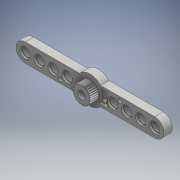
# Autodesk Inventor part: led-prop
Saved by Autodesk Inventor 2016 (Build 200138000, 138)
## iProperties
Created: 2016-11-01
Part Number: led-prop
Material: Generic
Document SubType Name: Modeling
Designer: Matt Ruffner
Density: 1 g/cm^3
Appearance: Default
Author: Matt Ruffner
Autodesk Inventor part; units mm, degrees
ref_plane "YZ Plane" through (0, 0, 0) normal (1, 0, 0) x (0, 1, 0)
ref_plane "XZ Plane" through (0, 0, 0) normal (0, 1, 0) x (-1, 0, 0)
ref_plane "XY Plane" through (0, 0, 0) normal (0, 0, 1) x (1, 0, 0)
sketch "Sketch1" plane through (0, 0, 0) normal (0, 1, 0) x (-1, 0, 0)
  circle A0 centre (24.5, 0) radius 5.05
  circle A1 centre (39.5, 0) radius 5.05
  circle A2 centre (54.5, 0) radius 5.05
  circle A3 centre (69.5, 0) radius 5.05
  circle A4 centre (-69.5, 0) radius 5.05
  circle A5 centre (-54.5, 0) radius 5.05
  circle A6 centre (-39.5, 0) radius 5.05
  circle A7 centre (-24.5, 0) radius 5.05
  line L0 (69.5, -10) -> (11.1803, -10)
  line L1 (69.5, 10) -> (11.1803, 10)
  arc A8 (69.5, -10) -> (69.5, 10) centre (69.5, 0) ccw
  line L2 (-69.5, -10) -> (-11.1803, -10)
  arc A9 (-69.5, 10) -> (-69.5, -10) centre (-69.5, 0) ccw
  line L3 (-69.5, 10) -> (-11.1803, 10)
  arc A10 (11.1803, 10) -> (-11.1803, 10) centre (0, 0) ccw
  arc A11 (-11.1803, -10) -> (11.1803, -10) centre (0, 0) ccw
  dimension "d1" = 10.1
  dimension "d2" = 10.1
  dimension "d3" = 10.1
  dimension "d4" = 10.1
  dimension "d5" = 24.5
  dimension "d6" = 15
  dimension "d7" = 15
  dimension "d8" = 15
  dimension "d11" = 360
  dimension "d16" = 360
  constraints: 12 centre point, 8 end point, 8 point on circle, 2 coincident, 2 horizontal, 34 other
  measures "d1" diameter of A0
  measures "d2" diameter of A1
  measures "d3" diameter of A2
  measures "d4" diameter of A3
  measures "d5" distance of A0.centre point (0, 0)
  measures "d6" distance of A1.centre A0.centre
  measures "d7" distance of A2.centre A1.centre
  measures "d8" distance of A3.centre A2.centre
extrude "Extrusion1" add sketch "Sketch1" along normal blind 9
sketch "Sketch2" plane through (0, 0, 0) normal (0, -1, 0) x (1, 0, 0)
  circle A0 centre (-69.5, 0) radius 5.05 projected
  circle A1 centre (-54.5, 0) radius 5.05 projected
  circle A2 centre (-39.5, 0) radius 5.05 projected
  circle A3 centre (-24.5, 0) radius 5.05 projected
  circle A4 centre (24.5, 0) radius 5.05 projected
  circle A5 centre (39.5, 0) radius 5.05 projected
  circle A6 centre (54.5, 0) radius 5.05 projected
  circle A7 centre (69.5, 0) radius 5.05 projected
  circle A8 centre (-69.5, 0) radius 5.6
  circle A9 centre (-54.5, 0) radius 5.6
  circle A10 centre (-39.5, 0) radius 5.6
  circle A11 centre (-24.5, 0) radius 5.6
  circle A12 centre (24.5, 0) radius 5.6
  circle A13 centre (39.5, 0) radius 5.6
  circle A14 centre (54.5, 0) radius 5.6
  circle A15 centre (69.5, 0) radius 5.6
  point P0 (0, 0)
  dimension "d20" = 11.2
  dimension "d21" = 11.2
  dimension "d22" = 11.2
  dimension "d23" = 11.2
  dimension "d24" = 11.2
  dimension "d25" = 11.2
  dimension "d26" = 11.2
  dimension "d27" = 11.2
  constraints: 8 centre point, 8 coincident
  measures "d20" diameter of A8
  measures "d21" diameter of A9
  measures "d22" diameter of A10
  measures "d23" diameter of A11
  measures "d24" diameter of A12
  measures "d25" diameter of A13
  measures "d26" diameter of A14
  measures "d27" diameter of A15
extrude "Extrusion2" cut sketch "Sketch2" against normal blind 2
sketch "Sketch4" plane through (0, 0, 0) normal (0, -1, 0) x (1, 0, 0)
  circle A0 centre (0, 0) radius 4.1
  circle A1 centre (0, 0) radius 9.75
  line L0 (0.0369, 9.7499) -> (-0.7015, 8.471)
  line L1 (0.0369, 9.7499) -> (1.3056, 9.7499) construction
  line L2 (0.0369, 9.7499) -> (0.7792, 8.4642)
  line L3 (0.0369, 9.7499) -> (1.4839, 9.7499) construction
  line L4 (-1.8659, 9.5698) -> (-2.3406, 8.1714)
  line L5 (-1.8659, 9.5698) -> (-0.887, 8.4536)
  line L6 (-3.697, 9.0219) -> (-3.8898, 7.5577)
  line L7 (-3.697, 9.0219) -> (-2.5192, 8.1181)
  line L8 (-5.3861, 8.1273) -> (-5.2895, 6.6537)
  line L9 (-5.3861, 8.1273) -> (-4.0546, 7.4706)
  line L10 (-6.8681, 6.9203) -> (-6.4859, 5.4939)
  line L11 (-6.8681, 6.9203) -> (-5.4341, 6.5361)
  line L12 (-8.0863, 5.4475) -> (-7.4331, 4.123)
  line L13 (-8.0863, 5.4475) -> (-6.6048, 5.3504)
  line L14 (-8.9936, 3.7652) -> (-8.0946, 2.5936)
  line L15 (-8.9936, 3.7652) -> (-7.5217, 3.959)
  line L16 (-9.5554, 1.9383) -> (-8.4451, 0.9646)
  line L17 (-9.5554, 1.9383) -> (-8.1496, 2.4155)
  line L18 (-9.7499, 0.0369) -> (-8.471, -0.7015)
  line L19 (-9.7499, 0.0369) -> (-8.4642, 0.7792)
  line L20 (-9.5698, -1.8659) -> (-8.1714, -2.3406)
  line L21 (-9.5698, -1.8659) -> (-8.4536, -0.887)
  line L22 (-9.0219, -3.697) -> (-7.5577, -3.8898)
  line L23 (-9.0219, -3.697) -> (-8.1181, -2.5192)
  line L24 (-8.1273, -5.3861) -> (-6.6537, -5.2895)
  line L25 (-8.1273, -5.3861) -> (-7.4706, -4.0546)
  line L26 (-6.9203, -6.8681) -> (-5.4939, -6.4859)
  line L27 (-6.9203, -6.8681) -> (-6.5361, -5.4341)
  line L28 (-5.4475, -8.0863) -> (-4.123, -7.4331)
  line L29 (-5.4475, -8.0863) -> (-5.3504, -6.6048)
  line L30 (-3.7652, -8.9936) -> (-2.5936, -8.0946)
  line L31 (-3.7652, -8.9936) -> (-3.959, -7.5217)
  line L32 (-1.9383, -9.5554) -> (-0.9646, -8.4451)
  line L33 (-1.9383, -9.5554) -> (-2.4155, -8.1496)
  line L34 (-0.0369, -9.7499) -> (0.7015, -8.471)
  line L35 (-0.0369, -9.7499) -> (-0.7792, -8.4642)
  line L36 (1.8659, -9.5698) -> (2.3406, -8.1714)
  line L37 (1.8659, -9.5698) -> (0.887, -8.4536)
  line L38 (3.697, -9.0219) -> (3.8898, -7.5577)
  line L39 (3.697, -9.0219) -> (2.5192, -8.1181)
  line L40 (5.3861, -8.1273) -> (5.2895, -6.6537)
  line L41 (5.3861, -8.1273) -> (4.0546, -7.4706)
  line L42 (6.8681, -6.9203) -> (6.4859, -5.4939)
  line L43 (6.8681, -6.9203) -> (5.4341, -6.5361)
  line L44 (8.0863, -5.4475) -> (7.4331, -4.123)
  line L45 (8.0863, -5.4475) -> (6.6048, -5.3504)
  line L46 (8.9936, -3.7652) -> (8.0946, -2.5936)
  line L47 (8.9936, -3.7652) -> (7.5217, -3.959)
  line L48 (9.5554, -1.9383) -> (8.4451, -0.9646)
  line L49 (9.5554, -1.9383) -> (8.1496, -2.4155)
  line L50 (9.7499, -0.0369) -> (8.471, 0.7015)
  line L51 (9.7499, -0.0369) -> (8.4642, -0.7792)
  line L52 (9.5698, 1.8659) -> (8.1714, 2.3406)
  line L53 (9.5698, 1.8659) -> (8.4536, 0.887)
  line L54 (9.0219, 3.697) -> (7.5577, 3.8898)
  line L55 (9.0219, 3.697) -> (8.1181, 2.5192)
  line L56 (8.1273, 5.3861) -> (6.6537, 5.2895)
  line L57 (8.1273, 5.3861) -> (7.4706, 4.0546)
  line L58 (6.9203, 6.8681) -> (5.4939, 6.4859)
  line L59 (6.9203, 6.8681) -> (6.5361, 5.4341)
  line L60 (5.4475, 8.0863) -> (4.123, 7.4331)
  line L61 (5.4475, 8.0863) -> (5.3504, 6.6048)
  line L62 (3.7652, 8.9936) -> (2.5936, 8.0946)
  line L63 (3.7652, 8.9936) -> (3.959, 7.5217)
  line L64 (1.9383, 9.5554) -> (0.9646, 8.4451)
  line L65 (1.9383, 9.5554) -> (2.4155, 8.1496)
  arc A2 (-3.8898, 7.5577) -> (-4.0546, 7.4706) centre (0, 0) ccw
  arc A3 (-5.2895, 6.6537) -> (-5.4341, 6.5361) centre (0, 0) ccw
  arc A4 (-6.4859, 5.4939) -> (-6.6048, 5.3504) centre (0, 0) ccw
  arc A5 (-7.4331, 4.123) -> (-7.5217, 3.959) centre (0, 0) ccw
  arc A6 (-8.0946, 2.5936) -> (-8.1496, 2.4155) centre (0, 0) ccw
  arc A7 (-8.4451, 0.9646) -> (-8.4642, 0.7792) centre (0, 0) ccw
  arc A8 (-8.471, -0.7015) -> (-8.4536, -0.887) centre (0, 0) ccw
  arc A9 (-8.1714, -2.3406) -> (-8.1181, -2.5192) centre (0, 0) ccw
  arc A10 (-7.5577, -3.8898) -> (-7.4706, -4.0546) centre (0, 0) ccw
  arc A11 (-6.6537, -5.2895) -> (-6.5361, -5.4341) centre (0, 0) ccw
  arc A12 (-5.4939, -6.4859) -> (-5.3504, -6.6048) centre (0, 0) ccw
  arc A13 (-2.3406, 8.1714) -> (-2.5192, 8.1181) centre (0, 0) ccw
  arc A14 (-0.7015, 8.471) -> (-0.887, 8.4536) centre (0, 0) ccw
  arc A15 (0.9646, 8.4451) -> (0.7792, 8.4642) centre (0, 0) ccw
  arc A16 (2.5936, 8.0946) -> (2.4155, 8.1496) centre (0, 0) ccw
  arc A17 (4.123, 7.4331) -> (3.959, 7.5217) centre (0, 0) ccw
  arc A18 (5.4939, 6.4859) -> (5.3504, 6.6048) centre (0, 0) ccw
  arc A19 (6.6537, 5.2895) -> (6.5361, 5.4341) centre (0, 0) ccw
  arc A20 (7.5577, 3.8898) -> (7.4706, 4.0546) centre (0, 0) ccw
  arc A21 (8.1714, 2.3406) -> (8.1181, 2.5192) centre (0, 0) ccw
  arc A22 (8.471, 0.7015) -> (8.4536, 0.887) centre (0, 0) ccw
  arc A23 (8.4451, -0.9646) -> (8.4642, -0.7792) centre (0, 0) ccw
  arc A24 (8.0946, -2.5936) -> (8.1496, -2.4155) centre (0, 0) ccw
  arc A25 (7.4331, -4.123) -> (7.5217, -3.959) centre (0, 0) ccw
  arc A26 (6.4859, -5.4939) -> (6.6048, -5.3504) centre (0, 0) ccw
  arc A27 (5.2895, -6.6537) -> (5.4341, -6.5361) centre (0, 0) ccw
  arc A28 (3.8898, -7.5577) -> (4.0546, -7.4706) centre (0, 0) ccw
  arc A29 (2.3406, -8.1714) -> (2.5192, -8.1181) centre (0, 0) ccw
  arc A30 (0.7015, -8.471) -> (0.887, -8.4536) centre (0, 0) ccw
  arc A31 (-0.9646, -8.4451) -> (-0.7792, -8.4642) centre (0, 0) ccw
  arc A32 (-4.123, -7.4331) -> (-3.959, -7.5217) centre (0, 0) ccw
  arc A33 (-2.5936, -8.0946) -> (-2.4155, -8.1496) centre (0, 0) ccw
  dimension "d42" = 19.5
  dimension "d41" = 8.2
  dimension "d44" = 120
  dimension "d45" = 60
  dimension "d48" = 360
  constraints: 132 end point, 2 coincident, 2 horizontal, 1 centre point, 261 other
  measures "d41" diameter of A0
  measures "d44" angle of L0 L1
  measures "d45" angle of L2 L3
extrude "Extrusion3" add sketch "Sketch4" along normal blind 9 contours L53 A22 L50 L51 A23 L48 L49 A24 L46 L47 A25 L44 L45 A26 L42 L43 A27 L40 L41 A28 L38 L39 A29 L36 L37 A30 L34 L35 A31 L32 L33 A33 L30 L31 A32 L28 L29 A12 L26 L27 A11 L24 L25 A10 L22 L23 A9 L20 L21 A8 L18 L19 A7 L16 L17 A6 L14 L15 A5 L12 L13 A4 L10 L11 A3 L8 L9 A2 L6 L7 A13 L4 L5 A14 L0 L2 A15 L64 L65 A16 L62 L63 A17 L60 L61 A18 L58 L59 A19 L56 L57 A20 L54 L55 A21 L52
sketch "Sketch5" plane through (0, 0, 0) normal (0, -1, 0) x (1, 0, 0)
  line L0 (10.1249, 7.4) -> (18.5249, 7.4)
  line L1 (18.5249, 7.4) -> (18.5249, -7.4)
  line L2 (18.5249, -7.4) -> (10.1249, -7.4)
  line L3 (10.1249, -7.4) -> (10.1249, 7.4)
  line L4 (69.5, 10) -> (11.1803, 10) projected
  circle A0 centre (14.3249, -4.45) radius 1.6
  point P0 (0, 0)
  point P1 (9.7499, -0.0369)
  dimension "d52" = 8.4
  dimension "d53" = 14.8
  dimension "d54" = 2.6
  dimension "d55" = 0.375
  dimension "d56" = 3.2
  dimension "d57" = 2.95
  constraints: 8 end point, 2 parallel, 1 centre point, 1 horizontal, 1 perpendicular
  measures "d52" distance of L1.end L2.end
  measures "d53" distance of L0.end L1.end
  measures "d54" distance between parallel lines of L4 L0
  measures "d55" distance from line of point (9.75, -0.037) L3
  measures "d56" diameter of A0
  measures "d57" distance from line of L2 A0.centre
extrude "Extrusion4" cut sketch "Sketch5" against normal blind 3.5
sketch "Sketch6" plane through (0, 0, 0) normal (0, -1, 0) x (1, 0, 0)
  circle A0 centre (32, 6) radius 2
  circle A1 centre (24.5, 0) radius 5.05 projected
  circle A2 centre (-32, -6) radius 2
  circle A3 centre (-24.5, 0) radius 5.05 projected
  point P0 (0, 0)
  dimension "d60" = 4
  dimension "d61" = 7.5
  dimension "d62" = 6
  dimension "d63" = 4
  dimension "d64" = 7.5
  dimension "d65" = 6
  constraints: 2 centre point
  measures "d60" diameter of A0
  measures "d61" horizontal distance of A1.centre A0.centre
  measures "d62" vertical distance of A1.centre A0.centre
  measures "d63" diameter of A2
  measures "d64" horizontal distance of A3.centre A2.centre
  measures "d65" vertical distance of A3.centre A2.centre
extrude "Extrusion5" cut sketch "Sketch6" against normal through all contours A0 | A2
body "Solid1"
